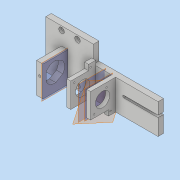
# Autodesk Inventor part: cellSTORM_inverted_Laser_10x_laserscanner_left_v2
Saved by Autodesk Inventor 2019.4 (Build 234330000, 330)
## iProperties
Created: 2020-11-05
Part Number: cellSTORM_inverted_Laser_10x_laserscanner_left_v2
Material: Generic
Document SubType Name: Modeling
Designer: diederichbenedict
Density: 1 g/cm^3
Appearance: Default
Author: diederichbenedict
Autodesk Inventor part; units mm, degrees
ref_plane "YZ Plane" through (0, 0, 0) normal (1, 0, 0) x (0, 1, 0)
ref_plane "XZ Plane" through (0, 0, 0) normal (0, 1, 0) x (-1, 0, 0)
ref_plane "XY Plane" through (0, 0, 0) normal (0, 0, 1) x (1, 0, 0)
ref_plane "Work Plane10" through (-44.5, -14.2241, 18.7548) normal (1, 0, 0) x (0, -0.9086751, 0.417504)
ref_plane "Work Plane11" through (-44.5, -8.5, 18.5) normal (-1, 0, 0) x (0, -1, 0)
sketch "Sketch9" plane through (-44.5, -8.5, 18.5) normal (-1, 0, 0) x (0, -1, 0)
  line L0 (16.8555, -12.7) -> (20, -12.7) construction
  circle A0 centre (17.5, -10) radius 1 construction
  circle A1 centre (11, 10.5) radius 1 construction
  circle A2 centre (-10.5, -5) radius 1 construction
  circle A3 centre (0, 0) radius 2.4142 construction
  line L1 (-15, 15) -> (15, 15) construction
  line L2 (16, -16) -> (-16, -16) construction
  line L3 (15, 15) -> (15, -15) construction
  line L4 (16, 16) -> (16, -16) construction
  line L5 (-16, -16) -> (-16, 16) construction
  line L6 (15, 15) -> (-16, 15)
  line L7 (-16, 15) -> (-16, -16.5)
  line L8 (-16, -16.5) -> (15, -16.5)
  line L9 (15, -16.5) -> (15, 15)
  circle A4 centre (11, 10.5) radius 0.9
  circle A5 centre (17.5, -10) radius 0.9
  circle A6 centre (-10.5, -5) radius 0.9
  circle A7 centre (0, 0) radius 9
  line L10 (15, -16.5) -> (22, -16.5)
  line L11 (22, -16.5) -> (22, -7.5)
  line L12 (22, -7.5) -> (15, -7.5)
  line L13 (15, -7.5) -> (15, -16.5)
  point P0 (-8.5, -18.5)
  dimension "d34" = 31.5
  dimension "d35" = 1.8
  dimension "d36" = 1.8
  dimension "d37" = 1.8
  dimension "d38" = 18
  dimension "d39" = 7
  dimension "d40" = 9
  constraints: 28 end point, 8 centre point, 5 horizontal, 4 coincident, 4 parallel, 3 vertical, 2 perpendicular, 1 point on line, 17 other
  measures "d34" distance of L7.end L6.end
  measures "d35" diameter of A4
  measures "d36" diameter of A5
  measures "d37" diameter of A6
  measures "d38" diameter of A7
  measures "d39" distance of L12.end L11.end
  measures "d40" distance of L11.end L10.end
extrude "Extrusion7" add sketch "Sketch9" against normal blind 5
ref_plane "Work Plane12" through (-127.4584, -23.859, -5) normal (0, 0, 1) x (1, 0, 0)
sketch "Sketch10" plane through (-44.5, -30.5, 2) normal (0, 0, -1) x (-1, 0, 0)
  line L0 (0, 0) -> (0, 38) projected
  line L1 (0, 38) -> (-5, 38) projected
  line L2 (-5, 0) -> (-5, 38) projected
  line L3 (0, 0) -> (-5, 0) projected
  circle A0 centre (-19, 22) radius 1.4
  circle A1 centre (-57, 22) radius 1.4
  line L4 (82.9584, 8.641) -> (82.9584, 51.641)
  line L5 (-58.4, 38) -> (82.9584, 38)
  line L6 (82.9584, 38) -> (82.9584, 0)
  line L7 (82.9584, 0) -> (-58.4, 0)
  line L8 (-58.4, 0) -> (-58.4, 38)
  line L9 (-63.3254, 22) -> (-14.2903, 22) construction
  line L10 (-61.7754, 20.45) -> (-15.8403, 20.45)
  line L11 (-15.8403, 23.55) -> (-61.7754, 23.55)
  arc A2 (-61.7754, 23.55) -> (-61.7754, 20.45) centre (-61.7754, 22) ccw
  arc A3 (-15.8403, 20.45) -> (-15.8403, 23.55) centre (-15.8403, 22) ccw
  point P0 (-44.5, 30.5)
  point P1 (-38.8079, 22)
  dimension "d43" = 3.1
  constraints: 18 end point, 6 point on circle, 4 centre point, 4 tangent, 3 parallel, 2 horizontal, 2 point on line, 1 midpoint, 1 perpendicular, 1 vertical, 6 other
  measures "d43" diameter of A3
extrude "Extrusion8" add sketch "Sketch10" along normal up to surface (7 mm away) contours L3 L2 L1 L0 | L0 L5 L4 L6 L7 | L7 L8 L10 A3 L11 L5 L2 | L8 L11 A3 L10
sketch "Sketch11" plane through (-44.5, -30.5, -5) normal (0, 0, -1) x (-1, 0, 0)
  circle A0 centre (-57, 22) radius 1.4 projected
  circle A1 centre (-19, 22) radius 1.4 projected
  line L0 (-61.4468, 22) -> (-14.0111, 22) construction
  line L1 (-60.0468, 20.6) -> (-15.4111, 20.6)
  line L2 (-15.4111, 23.4) -> (-60.0468, 23.4)
  arc A2 (-60.0468, 23.4) -> (-60.0468, 20.6) centre (-60.0468, 22) ccw
  arc A3 (-15.4111, 20.6) -> (-15.4111, 23.4) centre (-15.4111, 22) ccw
  point P0 (-44.5, 30.5)
  point P1 (-58.4, 22)
  point P2 (-37.729, 22)
  constraints: 8 end point, 6 point on circle, 4 tangent, 2 centre point, 2 point on line, 1 horizontal, 1 horizontal alignment, 1 midpoint, 1 parallel
extrude "Extrusion9" cut sketch "Sketch11" against normal through all contours A0 | A0 L2 A1 L1 | A0 L1 A2 L2 | L2 A3 L1 A1
ref_plane "Work Plane13" through (-99.5, -8.5, 18.5) normal (-1, 0, 0) x (0, 0, 1)
sketch "Sketch12" plane through (-99.5, -8.5, 18.5) normal (-1, 0, 0) x (0, 0, 1)
  circle A0 centre (0, 0) radius 10.125
  line L0 (-31.5, -12.684) -> (-23.5, -12.684)
  line L1 (-1.4, 6.6) -> (-6.6, 6.6)
  line L2 (-23.5, -22) -> (-23.5, 16) projected
  line L3 (-16.5, -22) -> (-23.5, -22) projected
  line L4 (-16.5, 16) -> (-16.5, -22) projected
  line L5 (-16.5, 16) -> (-23.5, 16) projected
  line L6 (15, 15) -> (15, -15)
  line L7 (-16.5, -22) -> (15, -22)
  line L8 (15, -22) -> (15, 16)
  line L9 (15, 16) -> (-16.5, 16)
  line L10 (-16.5, 16) -> (-16.5, -22)
  circle A1 centre (0, 0) radius 11.1
  line L11 (11.1, -5.0801) -> (11.1, 4.7426)
  line L12 (-1.1505, -12.1529) -> (-10.0048, -7.0409)
  line L13 (-10.0048, 7.0409) -> (-1.4428, 11.9842)
  arc A2 (-1.1505, -12.1529) -> (11.1, -5.0801) centre (0, 0) ccw
  arc A3 (11.1, 4.7426) -> (-1.4428, 11.9842) centre (0, 0) ccw
  arc A4 (-10.0048, 7.0409) -> (-10.0048, -7.0409) centre (0, 0) ccw
  point P0 (-18.5, 8.5)
  dimension "d51" = 60
  dimension "d52" = 60
  dimension "d73" = 22.2
  constraints: 20 end point, 6 point on circle, 5 centre point, 3 horizontal, 3 tangent, 2 parallel, 2 vertical, 1 perpendicular, 8 other
  measures "d51" angle of L12 L11
  measures "d52" angle of L13 L12
  measures "d73" diameter of A1
extrude "Extrusion10" add sketch "Sketch12" along normal blind 8 contours L4 L9 L8 L6 L7
sketch "Sketch13" plane through (-99.5, -30.5, 33.5) normal (0, 0, 1) x (1, 0, 0)
  line L0 (0, 38) -> (0, 0) projected
  line L1 (0, 38) -> (-8, 38) projected
  line L2 (-8, 0) -> (-8, 38) projected
  line L3 (0, 0) -> (-8, 0) projected
  line L4 (6.7208, 32.125) -> (-12.4892, 32.125)
  circle A0 centre (-4, 22.9829) radius 1.45
  point P0 (99.5, 30.5)
  dimension "d55" = 2.9
  constraints: 2 end point, 1 centre point, 1 horizontal, 2 other
  measures "d55" diameter of A0
extrude "Extrusion11" cut sketch "Sketch13" against normal blind 8 contours A0
sketch "Sketch14" plane through (-44.5, -30.5, 2) normal (0, 0, 1) x (1, 0, 0)
  circle A0 centre (-63, 55) radius 1.45
  circle A1 centre (-43, 55) radius 1.45
  line L0 (-55, 38) -> (-63, 38) projected
  line L1 (-82.9584, 38) -> (58.4, 38) projected
  line L2 (-82.9584, 38) -> (-22.9584, 38)
  line L3 (-22.9584, 38) -> (-22.9584, 60)
  line L4 (-22.9584, 60) -> (-82.9584, 60)
  line L5 (-82.9584, 60) -> (-82.9584, 38)
  point P0 (44.5, 30.5)
  dimension "d71" = 60
  dimension "d72" = 22
  constraints: 8 end point, 2 centre point, 2 parallel, 1 horizontal, 1 perpendicular, 4 other
  measures "d71" distance of L4.end L3.end
  measures "d72" distance of L3.end L2.end
ref_plane "Work Plane14" through (-127.4584, -23.859, -5) normal (0, 0, 1) x (1, 0, 0)
extrude "Extrusion12" add sketch "Sketch14" against normal up to surface (7 mm away)
sketch "Sketch15" plane through (-44.5, -30.5, 2) normal (0, 0, 1) x (1, 0, 0)
  line L0 (-82.9584, 0) -> (-63, 0) projected
  line L1 (-63, 0) -> (-63, 38) projected
  line L2 (-55, 38) -> (-63, 38) projected
  line L3 (-55, 38) -> (-55, 0) projected
  line L4 (-55, 0) -> (0, 0) projected
  line L5 (0, 0) -> (0, 38) projected
  line L6 (0, 38) -> (-22.9584, 38) projected
  line L7 (58.4, 20.6) -> (15.4111, 20.6) projected
  arc A0 (15.4111, 23.4) -> (15.4111, 20.6) centre (15.4111, 22) ccw projected
  line L8 (15.4111, 23.4) -> (58.4, 23.4) projected
  line L9 (58.4, 23.4) -> (58.4, 38) projected
  line L10 (5, 0) -> (5, 38) projected
  line L11 (5, 0) -> (58.4, 0) projected
  line L12 (58.4, 0) -> (58.4, 20.6) projected
  line L13 (-22.9584, 38) -> (-22.9584, 60) projected
  line L14 (-22.9584, 60) -> (-82.9584, 60) projected
  circle A1 centre (-63, 5) radius 1.45
  circle A2 centre (-43, 5) radius 1.45
  circle A3 centre (-43, 55) radius 1.45 projected
  circle A4 centre (-63, 55) radius 1.45 projected
  line L15 (-82.9584, 60) -> (-82.9584, 0) projected
  line L16 (58.4, 38) -> (5, 38) projected
  point P0 (44.5, 30.5)
  point P1 (-42.9584, 11.641)
  point P2 (-62.9584, 11.641)
  constraints: 2 centre point, 6 other
hole "Hole3" at (-107.5, -25.5, 2) at (-87.5, -25.5, 2) at (-107.5, 24.5, 2) at (-87.5, 24.5, 2) direction (0, 0, -1) diameter 3.3 end through all counterbore diameter 7 counterbore depth 3
ref_plane "Work Plane15" through (-53.5, -8.5, 18.5) normal (-1, 0, 0) x (0, 0, 1)
sketch "Sketch17" plane through (-44.5, -30.5, 2) normal (0, 0, 1) x (1, 0, 0)
  circle A0 centre (-63, 55) radius 3.5 projected
  arc A1 (-63, 8.5) -> (-63, 1.5) centre (-63, 5) ccw projected
  circle A2 centre (-43, 5) radius 3.5 projected
  circle A3 centre (-43, 55) radius 3.5 projected
  line L0 (-63, 0) -> (-63, 1.5) projected
  line L1 (58.4, 38) -> (5, 38) projected
  line L2 (-55, 38) -> (-55, 0) projected
  line L3 (-55, 0) -> (0, 0) projected
  line L4 (0, 0) -> (0, 38) projected
  line L5 (0, 38) -> (-22.9584, 38) projected
  line L6 (-22.9584, 38) -> (-22.9584, 60) projected
  line L7 (-22.9584, 60) -> (-82.9584, 60) projected
  line L8 (-82.9584, 60) -> (-82.9584, 0) projected
  line L9 (-82.9584, 0) -> (-63, 0) projected
  line L10 (5, 31) -> (5, 13) projected
  line L11 (0, 13) -> (0, 31) projected
  circle A4 centre (-10, 22) radius 0.5
  line L12 (58.4, 20.6) -> (15.4111, 20.6) projected
  arc A5 (15.4111, 23.4) -> (15.4111, 20.6) centre (15.4111, 22) ccw projected
  line L13 (15.4111, 23.4) -> (58.4, 23.4) projected
  line L14 (58.4, 23.4) -> (58.4, 38) projected
  line L15 (5, 0) -> (5, 38) projected
  line L16 (5, 0) -> (58.4, 0) projected
  line L17 (58.4, 0) -> (58.4, 20.6) projected
  line L18 (-55, 38) -> (-63, 38) projected
  line L19 (-63, 8.5) -> (-63, 38) projected
  point P0 (44.5, 30.5)
  dimension "d78" = 1
  dimension "d85" = 10
  constraints: 1 centre point
  measures "d78" diameter of A4
  measures "d85" distance from line of L4 A4.centre
extrude "Extrusion14" cut sketch "Sketch17" against normal blind 10 contours A4
pattern_circular "Circular Pattern1" count 2 over 360 about axis through (-54.5, -8.5, 2) along (0, 0, -1) of "Extrusion7"
body "Solid2"
